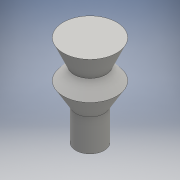
# Autodesk Inventor part: drive-pulley
Saved by Autodesk Inventor 2016 (Build 200138000, 138)
## iProperties
Created: 2016-11-04
Part Number: drive-pulley
Material: Generic
Document SubType Name: Modeling
Designer: Matt Ruffner
Density: 1 g/cm^3
Appearance: Default
Author: Matt Ruffner
Autodesk Inventor part; units mm, degrees
ref_plane "YZ Plane" through (0, 0, 0) normal (1, 0, 0) x (0, 1, 0)
ref_plane "XZ Plane" through (0, 0, 0) normal (0, 1, 0) x (-1, 0, 0)
ref_plane "XY Plane" through (0, 0, 0) normal (0, 0, 1) x (1, 0, 0)
sketch "Sketch1" plane through (0, 0, 0) normal (1, 0, 0) x (0, 1, 0)
  line L0 (0, 0) -> (5, 0)
  line L1 (0, 0) -> (0, -17)
  line L2 (0, -17) -> (2.65, -17)
  line L3 (2.65, -17) -> (2.65, -11)
  line L4 (3, -4.5) -> (5, 0)
  line L5 (5, -7) -> (3, -4.5)
  line L6 (2.65, -11) -> (5, -7)
  dimension "d1" = 17
  dimension "d2" = 2.65
  dimension "d3" = 6
  dimension "d11" = 5
  dimension "d12" = 3
  dimension "d13" = 5
  dimension "d14" = 4
  constraints: 14 end point, 2 perpendicular, 1 horizontal, 1 vertical
  measures "d1" distance of L0.start L1.end
  measures "d2" distance of L1.end L2.end
  measures "d3" distance of L2.end L3.end
  measures "d11" distance of L0.start L0.end
  measures "d12" distance from line of L1 L4.start
  measures "d13" distance from line of L1 L5.start
  measures "d14" vertical distance of L3.end L5.start
revolve "Revolution1" add sketch "Sketch1" angle 360 about axis through (0, 0, 0) along (0, 0, -1)
sketch "Sketch2" plane through (0, 0, -17) normal (0, 0, -1) x (-1, 0, 0)
  arc A0 (1.2369, -0.975) -> (-1.2369, -0.975) centre (0, 0) ccw
  line L0 (-1.9022, -0.975) -> (1.9927, -0.975)
  dimension "d7" = 3.15
  dimension "d8" = 2.55
  constraints: 2 end point, 2 point on circle, 2 point on line, 1 centre point, 1 coincident, 1 horizontal
  measures "d7" diameter of A0
extrude "Extrusion1" cut sketch "Sketch2" against normal blind 7
body "Solid1"
